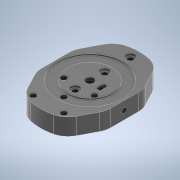
# Autodesk Inventor part: Platform
Saved by Autodesk Inventor 2022 (Build 260153000, 153)
## iProperties
Created: 2022-03-02
Part Number: Platform
Material: Genérico
Document SubType Name: Modeling
Designer: JK
Density: 1 g/cm^3
Appearance: Suave - Negro
Author: JK
Autodesk Inventor part; units mm, degrees
ref_plane "YZ Plane" through (0, 0, 0) normal (1, 0, 0) x (0, 1, 0)
ref_plane "XZ Plane" through (0, 0, 0) normal (0, 1, 0) x (-1, 0, 0)
ref_plane "XY Plane" through (0, 0, 0) normal (0, 0, 1) x (1, 0, 0)
sketch "Boceto1" plane through (0, 0, 0) normal (0, 1, 0) x (-1, 0, 0)
  circle A0 centre (0, 0) radius 19.876
  circle A1 centre (0, 0) radius 32.85
  circle A2 centre (0, 0) radius 50
  dimension "d0" = 65.7
  dimension "d1" = 100
  constraints: 3 centre point, 3 coincident
  measures "d0" diameter of A1
  measures "d1" diameter of A2
extrude "Extrusión1" add sketch "Boceto1" along normal blind 17 contours A0 | A1 | A2
sketch "Boceto2" plane through (0, 17, 0) normal (0, 1, 0) x (1, 0, 0)
  circle A0 centre (0, 0) radius 32.875
  circle A1 centre (0, 0) radius 22.45
  dimension "d4" = 65.75
  dimension "d5" = 44.9
  constraints: 2 centre point, 2 coincident
  measures "d4" diameter of A0
  measures "d5" diameter of A1
extrude "Extrusión2" cut sketch "Boceto2" against normal blind 1.4
sketch "Boceto3" plane through (0, 17, 0) normal (0, 1, 0) x (1, 0, 0)
  circle A0 centre (0, 0) radius 22.45 projected
extrude "Extrusión3" add sketch "Boceto3" along normal blind 1
sketch "Boceto4" plane through (0, 18, 0) normal (0, 1, 0) x (1, 0, 0)
  circle A0 centre (0, 0) radius 4
  line L0 (3, -2.6458) -> (3, 2.6458)
  dimension "d11" = 8
  dimension "d12" = 3
  constraints: 2 end point, 2 point on circle, 1 centre point, 1 coincident, 1 vertical
  measures "d11" diameter of A0
  measures "d12" distance from line of point (0, 0) L0
extrude "Extrusión4" cut sketch "Boceto4" against normal through all contours L0 A0 picked at (-0.1458, -1.2472)
sketch "Boceto5" plane through (0, 18, 0) normal (0, 1, 0) x (1, 0, 0)
  arc A0 (3, 2.6458) -> (3, -2.6458) centre (0, 0) ccw projected
  line L0 (3, 2.6458) -> (3, -2.6458) projected
  arc A1 (3.1, 2.6833) -> (3.1, -2.6833) centre (0, 0) ccw
  line L1 (3.1, 2.6833) -> (3.1, -2.6833)
  dimension "d15" = 0.1
  constraints: 2 end point, 2 point on circle, 1 centre point, 1 other
  measures "d15" radial gap between concentric circles of A1 A0
extrude "Extrusión5" cut sketch "Boceto5" against normal through all contours L0 A0 | L1 A1
sketch "Boceto6" plane through (0, 0, 0) normal (0, -1, 0) x (1, 0, 0)
  line L0 (-35, 64.067) -> (35, 64.067)
  line L1 (35, 64.067) -> (35, -64.067)
  line L2 (35, -64.067) -> (-35, -64.067)
  line L3 (-35, -64.067) -> (-35, 64.067)
  line L4 (-35, 64.067) -> (35, -64.067) construction
  line L5 (35, 64.067) -> (-35, -64.067) construction
  arc A0 (3.1, 2.6833) -> (3.1, -2.6833) centre (0, 0) ccw projected
  line L6 (3.1, 2.6833) -> (3.1, -2.6833) projected
  circle A1 centre (0, 0) radius 50 projected
  point P0 (0, 0)
  point P1 (-35, 35.7071)
  point P2 (-35, -35.7071)
  point P3 (35, 35.7071)
  point P4 (35, -35.7071)
  dimension "d19" = 70
  constraints: 12 end point, 3 midpoint, 2 parallel, 1 coincident, 1 horizontal, 1 perpendicular
  measures "d19" distance of L1.end L2.end
extrude "Extrusión6" cut sketch "Boceto6" against normal through all contours L3 A1 | A1 L1
chamfer "Chaflán1" distance 17 angle 45 4 edges at (-35, 8.5, 35.7071) (-35, 8.5, -35.7071) (35, 8.5, -35.7071) (35, 8.5, 35.7071)
fillet "Empalme2" radius 20 8 edges at (-21.0133, 8.5, 45.3701) (-35, 8.5, 18.7071) (-35, 8.5, -18.7071) (-21.0133, 8.5, -45.3701) (21.0133, 8.5, -45.3701) (35, 8.5, -18.7071) (35, 8.5, 18.7071) (21.0133, 8.5, 45.3701)
sketch "Boceto8" plane through (0, 18, 0) normal (0, 1, 0) x (1, 0, 0)
  arc A0 (3.1, 2.6833) -> (3.1, -2.6833) centre (0, 0) ccw projected
  line L0 (3.1, 2.6833) -> (3.1, -2.6833) projected
sketch "Boceto9" plane through (0, 17, 0) normal (0, 1, 0) x (1, 0, 0)
  circle A0 centre (0, 41) radius 2.7
  circle A1 centre (0, 15) radius 2.7
  circle A2 centre (0, -15) radius 2.7
  point P0 (0, 0)
  dimension "d30" = 5.4
  dimension "d31" = 5.4
  dimension "d32" = 15
  dimension "d33" = 26
  dimension "d45" = 15
  constraints: 3 centre point, 1 equal radius
  measures "d30" diameter of A0
  measures "d31" diameter of A1
  measures "d32" distance of A1.centre point (0, 0)
  measures "d33" distance of A1.centre A0.centre
  measures "d45" distance of A2.centre point (0, 0)
extrude "Extrusión8" cut sketch "Boceto9" along normal blind 15 and the other way blind 27.75
sketch "Boceto13" plane through (0, 17, 0) normal (0, 1, 0) x (1, 0, 0)
  circle A0 centre (0, 41) radius 2.7 projected
  circle A1 centre (0, 41) radius 4.6
  circle A2 centre (0, 15) radius 2.7 projected
  circle A3 centre (0, 15) radius 4.6
  circle A4 centre (0, -15) radius 2.7 projected
  circle A5 centre (0, -15) radius 4.6
  point P0 (0, 0)
  dimension "d38" = 9.2
  dimension "d39" = 9.2
  constraints: 3 centre point, 3 coincident, 1 equal radius
  measures "d38" diameter of A1
  measures "d39" diameter of A3
extrude "Extrusión9" cut sketch "Boceto13" along normal blind 2 and the other way blind 2 contours A0 | A1 | A3 | A4 | A5
sketch "Boceto14" plane through (0, 18, 0) normal (0, 1, 0) x (1, 0, 0)
  circle A0 centre (0, 0) radius 9
  dimension "d46" = 18
  constraints: 1 centre point, 1 coincident
  measures "d46" diameter of A0
extrude "Extrusión10" add sketch "Boceto14" along normal blind 2.5
sketch "Boceto15" plane through (0, 0, 0) normal (0, -1, 0) x (1, 0, 0)
  line L0 (3.1, -2.6833) -> (3.1, 2.6833) projected
  arc A0 (3.1, 2.6833) -> (3.1, -2.6833) centre (0, 0) ccw projected
extrude "Extrusión11" cut sketch "Boceto15" against normal through all
fillet "Empalme3" radius 2 1 edges at (-9, 18, 0)
sketch "Boceto16" plane through (0, 20.5, 0) normal (0, 1, 0) x (1, 0, 0)
  circle A0 centre (0, 0) radius 4.15
  constraints: 1 centre point, 1 coincident
extrude "Extrusión12" cut sketch "Boceto16" against normal blind 2
sketch "Boceto17" plane through (0, 18, 0) normal (0, 1, 0) x (1, 0, 0)
  arc A0 (1.9376, -10.828) -> (1.9376, 10.828) centre (0, 0) ccw projected
  arc A1 (-1.9376, -10.828) -> (1.9376, -10.828) centre (0, -15) ccw projected
  arc A2 (-1.9376, 10.828) -> (-1.9376, -10.828) centre (0, 0) ccw projected
  arc A3 (1.9376, 10.828) -> (-1.9376, 10.828) centre (0, 15) ccw projected
  circle A4 centre (0, 0) radius 22.45 projected
extrude "Extrusión13" cut sketch "Boceto17" against normal up to surface (1 mm away)
sketch "Boceto18" plane through (0, 17, 0) normal (0, 1, 0) x (1, 0, 0)
  circle A0 centre (0, 0) radius 13.4678
  constraints: 1 centre point, 1 coincident
extrude "Extrusión14" cut sketch "Boceto18" along normal blind 17.5
sketch "Boceto19" plane through (0, 17, 0) normal (0, 1, 0) x (1, 0, 0)
  circle A0 centre (0, 0) radius 4.15
  constraints: 1 centre point, 1 coincident
extrude "Extrusión15" cut sketch "Boceto19" against normal blind 3
sketch "Boceto20" plane through (0, 17, 0) normal (0, 1, 0) x (1, 0, 0)
  circle A0 centre (-15.5, -42) radius 1.65
  point P0 (0, 0)
  point P1 (0, -26.5)
  dimension "d60" = 15.5
  dimension "d61" = 15.5
  dimension "d62" = 3.3
  dimension "d84" = 42
  constraints: 1 centre point, 1 vertical alignment
  measures "d60" horizontal distance of A0.centre point (0, -26.5)
  measures "d61" horizontal distance of A0.centre point (0, -26.5)
  measures "d62" diameter of A0
  measures "d84" vertical distance of A0.centre point (0, 0)
extrude "Extrusión16" cut sketch "Boceto20" against normal through all
sketch "Boceto21" plane through (0, 17, 0) normal (0, 1, 0) x (1, 0, 0)
  line L0 (14.0981, 4.05) -> (9.8981, 4.05)
  line L1 (9.8981, 4.05) -> (9.8981, -4.05)
  line L2 (9.8981, -4.05) -> (14.0981, -4.05)
  line L3 (14.0981, -4.05) -> (14.0981, 4.05)
  line L4 (14.0981, 4.05) -> (9.8981, -4.05) construction
  line L5 (9.8981, 4.05) -> (14.0981, -4.05) construction
  point P0 (0, 0)
  point P1 (11.9981, 0)
  dimension "d65" = 8.1
  dimension "d66" = 4.2
  constraints: 12 end point, 2 midpoint, 2 parallel, 1 horizontal, 1 perpendicular
  measures "d65" distance between parallel lines of L2 L0
  measures "d66" distance between parallel lines of L3 L1
extrude "Extrusión17" cut sketch "Boceto21" against normal blind 14
sketch "Boceto22" plane through (35, 0, 13.7798) normal (1, 0, 0) x (0, 0, -1)
  circle A0 centre (13.7798, 7.6) radius 2.7
  line L0 (17.8298, 3) -> (9.7298, 3) projected
  point P0 (13.7798, 0)
  point P1 (13.7798, 3)
  dimension "d69" = 5.4
  dimension "d70" = 4.6
  constraints: 1 centre point, 1 midpoint, 1 vertical alignment
  measures "d69" diameter of A0
  measures "d70" distance from line of L0 A0.centre
extrude "Extrusión18" cut sketch "Boceto22" against normal blind 35.25
sketch "Boceto23" plane through (0, 17, 0) normal (0, 1, 0) x (1, 0, 0)
  circle A0 centre (0, -26.5) radius 3
  circle A1 centre (-15.5, -42) radius 1.65 projected
  point P0 (0, 0)
  dimension "d73" = 15.5
  dimension "d74" = 15.5
  dimension "d81" = 6
  constraints: 1 centre point
  measures "d73" horizontal distance of A1.centre A0.centre
  measures "d74" horizontal distance of A1.centre A0.centre
  measures "d81" diameter of A0
extrude "Extrusión20" cut sketch "Boceto23" against normal through all contours A0
sketch "Boceto24" plane through (0, 17, 0) normal (0, 1, 0) x (1, 0, 0)
  circle A0 centre (-15.5, -42) radius 1.65 projected
  circle A1 centre (-15.5, -42) radius 3
  point P0 (0, 0)
  dimension "d78" = 6
  constraints: 1 centre point, 1 coincident
  measures "d78" diameter of A1
extrude "Extrusión19" cut sketch "Boceto24" against normal blind 4
pattern_circular "Patrón circular1" count 4 over 360 about axis through (0, 17, 26.5) along (0, 1, 0) of "Extrusión16", "Extrusión20", "Extrusión19"
